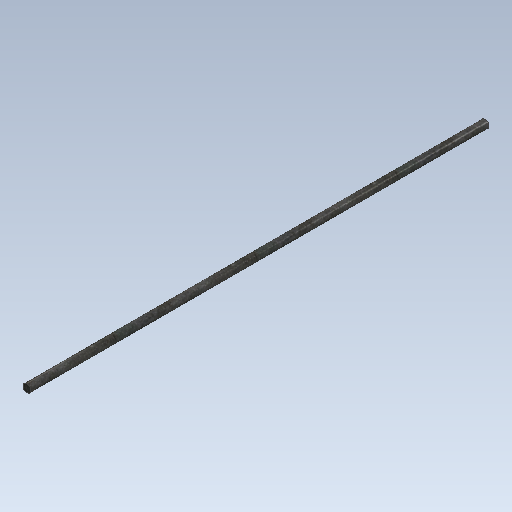
# Autodesk Inventor part: 0008-10-1008 Bara 10_V1
Saved by Autodesk Inventor 2020 (Build 240168000, 168)
## iProperties
Created: 2021-03-01
Part Number: 0008-10-1008 Bara 10_V1
Material: Steel
Document SubType Name: Modeling
Designer: Iulian Bors
Density: 7.85 g/cm^3
Appearance: Plate
Mass: 351.426 g
Surface Area: 180.642 cm^2
Volume: 44.7677 cm^3
Description: Bara 10
Author: Iulian Bors
Subject: 1008
Autodesk Inventor part; units mm, degrees
ref_plane "YZ Plane" through (0, 0, 0) normal (1, 0, 0) x (0, 1, 0)
ref_plane "XZ Plane" through (0, 0, 0) normal (0, 1, 0) x (-1, 0, 0)
ref_plane "XY Plane" through (0, 0, 0) normal (0, 0, 1) x (1, 0, 0)
sketch "Sketch1" plane through (0, 0, 0) normal (0, 0, 1) x (1, 0, 0)
  circle A0 centre (0, 0) radius 5
  dimension "d0" = 10
  constraints: 1 centre point, 1 coincident
  measures "d0" diameter of A0
extrude "Extrusion1" add sketch "Sketch1" along normal mid plane 570
body "Solid1"
